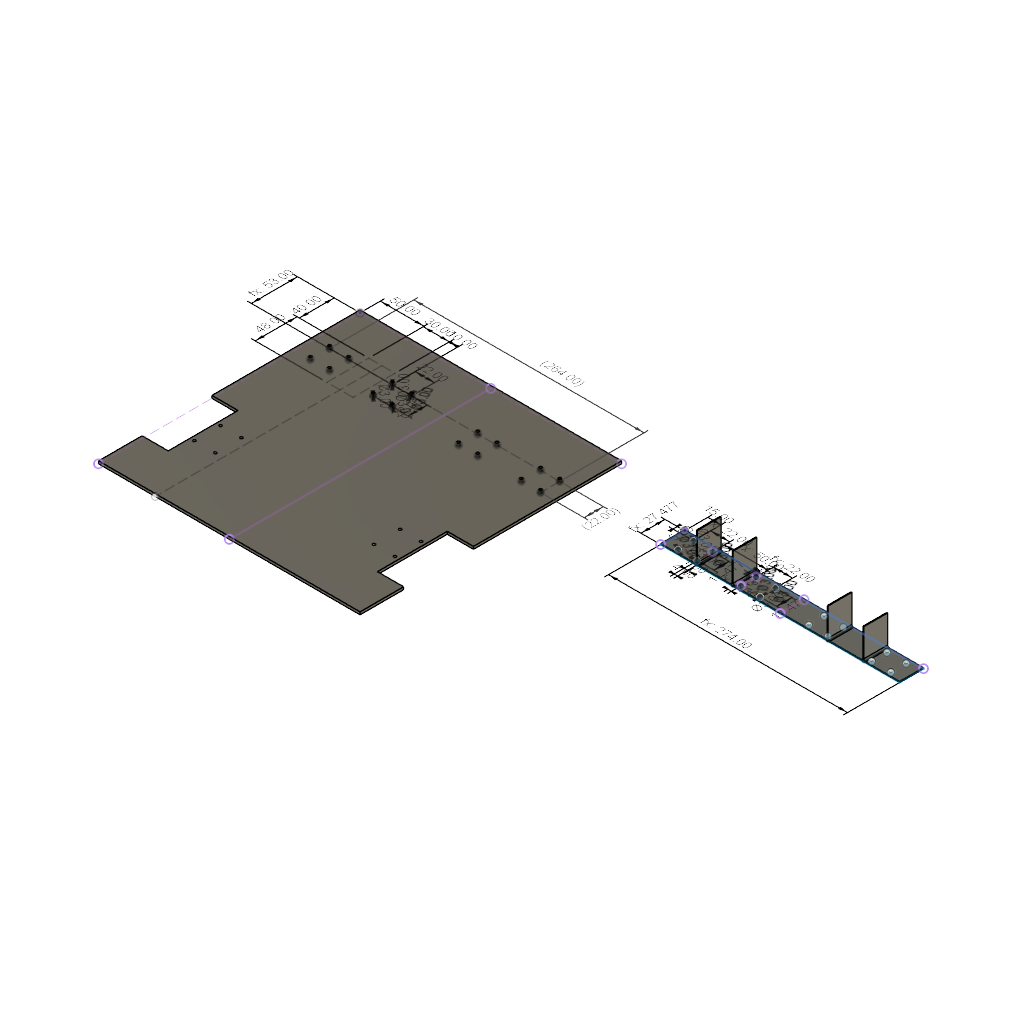
ZoMa Chassis v2.0 (Autodesk Fusion 360 design; units mm, degrees)
part number: 2026-08-13-13-10-42-406
Autodesk Fusion 360 part; units mm, degrees
sketch "Base Sheet" plane through (0, 0, 0) normal (0, 0, 1) x (1, 0, 0)
  line L0 (150, -150) -> (-150, -150)
  line L1 (-150, -150) -> (-150, 150)
  line L2 (-150, 150) -> (150, 150)
  line L3 (150, 150) -> (150, -150)
  line L4 (150, -150) -> (-150, 150) construction
  line L5 (-150, -150) -> (150, 150) construction
  dimension "d1" = 300
  dimension "d2" = 300
  constraint horizontal L0
  constraint perpendicular L0 L1
  constraint parallel L0 L2
  constraint parallel L1 L3
  constraint coincident L4 origin
  constraint coincident L5 origin
  measures "d1" distance of L1.end L2.end
  measures "d2" distance of L0.end L1.end
sketch "Rear Wheels Motors" plane through (0, 0, 0) normal (0, 0, 1) x (1, 0, 0)
  line L0 (-150, -20) -> (-120, -20)
  line L1 (-120, -20) -> (-120, -100)
  line L2 (-120, -100) -> (-150, -100)
  line L3 (-150, -100) -> (-150, -20)
  line L4 (150, -150) -> (-150, -150)
  line L5 (-150, -150) -> (-150, 150)
  line L6 (-115, -45) -> (-91, -45) construction
  line L7 (-91, -45) -> (-91, -75) construction
  line L8 (-91, -75) -> (-115, -75) construction
  line L9 (-115, -75) -> (-115, -45) construction
  circle A0 centre (-115, -45) radius 1.5
  circle A1 centre (-91, -45) radius 1.5
  circle A2 centre (-91, -75) radius 1.5
  circle A3 centre (-115, -75) radius 1.5
  line L10 (0, 150) -> (0, -150) construction
  circle A4 centre (115, -45) radius 1.5
  circle A5 centre (91, -45) radius 1.5
  circle A6 centre (91, -75) radius 1.5
  circle A7 centre (115, -75) radius 1.5
  line L11 (120, -20) -> (120, -100)
  line L12 (150, -20) -> (120, -20)
  line L13 (150, -100) -> (150, -20)
  line L14 (120, -100) -> (150, -100)
  dimension "d3" = 30
  dimension "d4" = 80
  dimension "d5" = 50
  dimension "d6" = 24
  dimension "d7" = 30
  dimension "d8" = 75
  dimension "d9" = 5
  dimension "d10" = 3
  dimension "d11" = 3
  dimension "d12" = 3
  dimension "d13" = 3
  constraint horizontal L0
  constraint vertical L1
  constraint horizontal L2
  constraint vertical L3
  constraint coincident L2.end L5
  constraint horizontal L6
  constraint vertical L7
  constraint horizontal L8
  constraint vertical L9
  constraint coincident L6.start L9.end
  constraint coincident L6.end L7.start
  constraint coincident L7.end L8.start
  constraint coincident L8.end L9.start
  constraint midpoint L4 L10.end
  constraint perpendicular L4 L10
  constraint symmetric L0.start L10 L12.start
  constraint symmetric L0.end L10 L11.start
  constraint symmetric L1.end L10 L11.end
  constraint symmetric L2.end L10 L13.start
  constraint symmetric A0 L10 A4
  constraint symmetric A1 L10 A5
  constraint symmetric A2 L10 A6
  constraint symmetric A3 L10 A7
  measures "d3" distance of L0.start L0.end
  measures "d4" distance of L0.start L2.end
  measures "d5" distance of L2 L4
  measures "d6" distance of L6.start L6.end
  measures "d7" distance of L6.start L8.end
  measures "d8" distance of L4 L8
  measures "d9" distance of L1 L9
  measures "d10" diameter of A0
  measures "d11" diameter of A1
  measures "d12" diameter of A2
  measures "d13" diameter of A3
sketch "Front Omni Wheels" plane through (0, 0, 0) normal (0, 0, 1) x (1, 0, 0)
  line L0 (-100, 110) -> (-70, 110) construction
  line L1 (-70, 110) -> (-70, 62) construction
  line L2 (-70, 62) -> (-100, 62) construction
  line L3 (-100, 62) -> (-100, 110) construction
  line L4 (-150, -150) -> (-150, 150) construction
  line L5 (-150, 150) -> (150, 150) construction
  line L6 (-85, 110) -> (-85, -150) construction
  line L7 (-60, 97) -> (-38, 97) construction
  line L8 (-38, 97) -> (-38, 75) construction
  line L9 (-38, 75) -> (-60, 75) construction
  line L10 (-60, 75) -> (-60, 97) construction
  circle A0 centre (-60, 97) radius 1.5
  circle A1 centre (-38, 97) radius 1.5
  circle A2 centre (-60, 75) radius 1.5
  circle A3 centre (-38, 75) radius 1.5
  circle A4 centre (-110, 97) radius 1.5
  circle A5 centre (-132, 97) radius 1.5
  circle A6 centre (-110, 75) radius 1.5
  circle A7 centre (-132, 75) radius 1.5
  line L11 (0, 150) -> (0, -150)
  circle A8 centre (38, 97) radius 1.5
  circle A9 centre (38, 75) radius 1.5
  circle A10 centre (60, 75) radius 1.5
  circle A11 centre (60, 97) radius 1.5
  circle A12 centre (110, 97) radius 1.5
  circle A13 centre (110, 75) radius 1.5
  circle A14 centre (132, 75) radius 1.5
  circle A15 centre (132, 97) radius 1.5
  line L12 (-132, 97) -> (132, 97) construction
  line L13 (132, 97) -> (132, 75) construction
  line L14 (252.4841, 119.672) -> (526.4841, 119.672)
  line L15 (526.4841, 119.672) -> (526.4841, 92.1946)
  line L16 (526.4841, 92.1946) -> (252.4841, 92.1946)
  line L17 (252.4841, 92.1946) -> (252.4841, 119.672)
  line L18 (267.4841, 114.672) -> (289.4841, 114.672) construction
  line L19 (289.4841, 114.672) -> (289.4841, 97.1946) construction
  line L20 (289.4841, 97.1946) -> (267.4841, 97.1946) construction
  line L21 (267.4841, 97.1946) -> (267.4841, 114.672) construction
  line L22 (361.4841, 114.672) -> (361.4841, 97.1946) construction
  line L23 (339.4841, 114.672) -> (361.4841, 114.672) construction
  line L24 (339.4841, 97.1946) -> (339.4841, 114.672) construction
  line L25 (361.4841, 97.1946) -> (339.4841, 97.1946) construction
  circle A16 centre (267.4841, 114.672) radius 1.5
  circle A17 centre (289.4841, 114.672) radius 1.5
  circle A18 centre (267.4841, 97.1946) radius 1.5
  circle A19 centre (289.4841, 97.1946) radius 1.5
  circle A20 centre (339.4841, 114.672) radius 1.5
  circle A21 centre (339.4841, 97.1946) radius 1.5
  circle A22 centre (361.4841, 114.672) radius 1.5
  circle A23 centre (361.4841, 97.1946) radius 1.5
  line L26 (389.4841, 119.672) -> (389.4841, 92.1946) construction
  circle A24 centre (511.4841, 114.672) radius 1.5
  circle A25 centre (489.4841, 114.672) radius 1.5
  circle A26 centre (511.4841, 97.1946) radius 1.5
  circle A27 centre (489.4841, 97.1946) radius 1.5
  circle A28 centre (439.4841, 114.672) radius 1.5
  circle A29 centre (417.4841, 114.672) radius 1.5
  circle A30 centre (439.4841, 97.1946) radius 1.5
  circle A31 centre (417.4841, 97.1946) radius 1.5
  dimension "d14" = 30
  dimension "d15" = 48
  dimension "d16" = 50
  dimension "d17" = 40
  dimension "d18" = 22
  dimension "d19" = 22
  dimension "d20" = 53
  dimension "d21" = 10
  dimension "d22" = 3
  dimension "d23" = 3
  dimension "d24" = 3
  dimension "d25" = 3
  dimension "d31" = 264
  dimension "d32" = 22
  dimension "d33" = 274
  dimension "d34" = 27.4774
  dimension "d41" = 22
  dimension "d42" = 17.4774
  dimension "d43" = 22
  dimension "d44" = 17.4774
  dimension "d45" = 50
  dimension "d46" = 3
  dimension "d47" = 3
  dimension "d48" = 3
  dimension "d49" = 3
  dimension "d50" = 3
  dimension "d51" = 3
  dimension "d52" = 3
  dimension "d53" = 3
  dimension "d54" = 15
  dimension "d55" = 5
  dimension "d56" = 5
  constraint horizontal L0
  constraint vertical L1
  constraint horizontal L2
  constraint vertical L3
  constraint midpoint L0 L6.start
  constraint perpendicular L2 L6
  constraint horizontal L7
  constraint vertical L8
  constraint horizontal L9
  constraint vertical L10
  constraint coincident L7.start L10.end
  constraint coincident L7.end L8.start
  constraint coincident L9.end L10.start
  constraint coincident L8.end L9.start
  constraint symmetric L6 A0 A4
  constraint symmetric L6 A1 A5
  constraint symmetric L6 A2 A6
  constraint symmetric L6 A3 A7
  constraint symmetric A0 L11 A11
  constraint symmetric A1 L11 A8
  constraint symmetric A2 L11 A10
  constraint symmetric A3 L11 A9
  constraint symmetric A4 L11 A12
  constraint symmetric A5 L11 A15
  constraint symmetric A6 L11 A13
  constraint symmetric A7 L11 A14
  constraint coincident A5.centre L12.start
  constraint coincident A15.centre L12.end
  constraint coincident A14.centre L13.end
  constraint horizontal L14
  constraint vertical L15
  constraint horizontal L16
  constraint vertical L17
  constraint horizontal L18
  constraint vertical L19
  constraint horizontal L20
  constraint vertical L21
  constraint horizontal L23
  constraint vertical L22
  constraint horizontal L25
  constraint vertical L24
  constraint coincident L18.start L21.end
  constraint coincident L18.end L19.start
  constraint coincident L20.end L21.start
  constraint coincident L19.end L20.start
  constraint coincident L23.start L24.end
  constraint coincident L24.start L25.end
  constraint coincident L22.start L23.end
  constraint coincident L22.end L25.start
  constraint midpoint L14 L26.start
  constraint midpoint L16 L26.end
  constraint symmetric A16 L26 A24
  constraint symmetric A17 L26 A25
  constraint symmetric A18 L26 A26
  constraint symmetric A19 L26 A27
  constraint symmetric A20 L26 A28
  constraint symmetric A21 L26 A30
  constraint symmetric A22 L26 A29
  constraint symmetric A23 L26 A31
  measures "d14" distance of L0.start L0.end
  measures "d15" distance of L0.start L2.end
  measures "d16" distance of L3 L4
  measures "d17" distance of L0 L5
  measures "d18" distance of L7.start L7.end
  measures "d19" distance of L7.start L9.end
  measures "d20" distance of L5 L7
  measures "d21" distance of L1 L10
  measures "d22" diameter of A0
  measures "d23" diameter of A1
  measures "d24" diameter of A2
  measures "d25" diameter of A3
  measures "d31" distance of A5.centre A15.centre
  measures "d32" distance of A15.centre A14.centre
  measures "d33" distance of L14.start L14.end
  measures "d34" distance of L14.start L16.end
  measures "d41" distance of L18.start L18.end
  measures "d42" distance of L18.end L19.end
  measures "d43" distance of L23.start L22.start
  measures "d44" distance of L22.start L22.end
  measures "d45" distance of L19 L24
  measures "d46" diameter of A16
  measures "d47" diameter of A17
  measures "d48" diameter of A18
  measures "d49" diameter of A19
  measures "d50" diameter of A20
  measures "d51" diameter of A21
  measures "d52" diameter of A22
  measures "d53" diameter of A23
  measures "d54" distance of L17 L18.start
  measures "d55" distance of L14 L18
  measures "d56" distance of L14 L23
extrude "Extrude1" add sketch "Front Omni Wheels" sketch "Base Sheet" along normal blind 3 contours A0 | A1 | A2 | A3 | A4 | A5 | A6 | A7 | A8 | A9 | A10 | A11 | A12 | A13 | A14 | A15 of sketch 2 makes body 1
extrude "Extrude2" cut sketch "Rear Wheels Motors" sketch "Front Omni Wheels" along normal blind 3 of sketch 2 contours A0 | A1 | A2 | A3 | A4 | A5 | A6 | A7 | A8 | A9 | A10 | A11 | A12 | A13 | A14 | A15 bodies 1
extrude "Extrude4" add sketch "Front Omni Wheels" along normal blind 1 separate body contours L14 L15 L16 L17 makes body 2
sketch "Sketch6" plane through (0, 0, 0) normal (0, 0, 1) x (1, 0, 0)
  line L0 (293.4841, 119.6622) -> (294.4841, 119.6622)
  line L1 (294.4841, 119.6622) -> (294.4841, 92.1847)
  line L2 (294.4841, 92.1847) -> (293.4841, 92.1847)
  line L3 (293.4841, 92.1847) -> (293.4841, 119.6622)
  line L4 (252.4841, 92.1946) -> (252.4841, 119.672)
  line L5 (334.4841, 119.672) -> (335.4841, 119.672)
  line L6 (335.4841, 119.672) -> (335.4841, 92.1946)
  line L7 (335.4841, 92.1946) -> (334.4841, 92.1946)
  line L8 (334.4841, 92.1946) -> (334.4841, 119.672)
  line L9 (252.4841, 119.672) -> (526.4841, 119.672)
  line L10 (339.4841, 97.1946) -> (339.4841, 114.672)
  line L11 (389.4841, 119.672) -> (389.4841, 92.1946)
  line L12 (485.4841, 92.1847) -> (485.4841, 119.6622)
  line L13 (484.4841, 119.6622) -> (484.4841, 92.1847)
  line L14 (444.4841, 92.1946) -> (444.4841, 119.672)
  line L15 (443.4841, 119.672) -> (443.4841, 92.1946)
  line L16 (443.4841, 92.1946) -> (444.4841, 92.1946)
  line L17 (443.4841, 119.672) -> (444.4841, 119.672)
  line L18 (484.4841, 119.6622) -> (485.4841, 119.6622)
  line L19 (485.4841, 92.1847) -> (484.4841, 92.1847)
  point P0 (289.4841, 114.672)
  dimension "d61" = 1
  dimension "d62" = 4
  dimension "d63" = 4
  constraint horizontal L0
  constraint vertical L1
  constraint horizontal L2
  constraint vertical L3
  constraint equal L1 L4
  constraint horizontal L5
  constraint vertical L6
  constraint horizontal L7
  constraint vertical L8
  constraint equal L4 L8
  constraint equal L2 L7
  constraint coincident L5.start L9
  constraint symmetric L0.start L11 L12.end
  constraint symmetric L0.end L11 L13.start
  constraint symmetric L1.end L11 L13.end
  constraint symmetric L2.end L11 L12.start
  constraint symmetric L5.start L11 L14.end
  constraint symmetric L5.end L11 L15.start
  constraint symmetric L6.end L11 L15.end
  constraint symmetric L7.end L11 L14.start
  measures "d61" distance of L1.end L2.end
  measures "d62" distance of L3 P0
  measures "d63" distance of L6 L10
extrude "Extrude5" add sketch "Sketch6" along normal blind 35 bodies 2
fillet "Fillet1" radius 2 8 edges at (335.4841, 105.9333, 1) (294.4841, 105.9284, 1) (485.4841, 105.9284, 1) (293.4841, 105.9284, 1) (334.4841, 105.9333, 1) (443.4841, 105.9333, 1) (484.4841, 105.9284, 1) (444.4841, 105.9333, 1) on bodies 2
equation "d8 = d5 + d4 / 2 - d7 / 2"
equation "d20 = d17 + d15 / 2 - d19 / 2"
equation "d33 = d31 + 10 mm"
equation "d34 = d42 + 10 mm"
equation "d36 = d32"
equation "d41 = d18"
equation "d43 = d18"
equation "d45 = d14 + d21 * 2"
equation "d56 = d55"
equation "d63 = d62"
